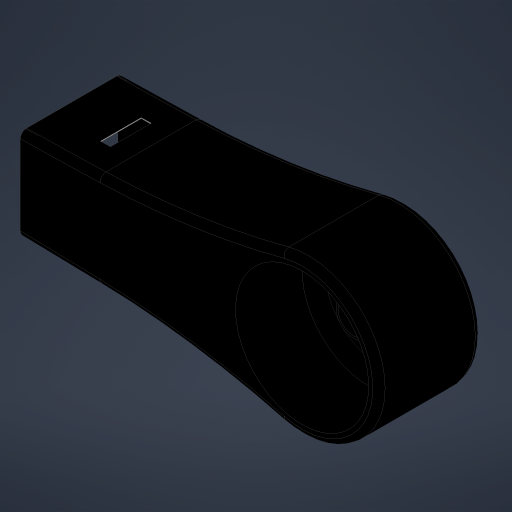
# Autodesk Inventor part: Arm
Saved by Autodesk Inventor 2023 (Build 270158000, 158)
## iProperties
Created: 2023-04-09
Part Number: Arm
Material: Generic
Document SubType Name: Modeling
Designer: vatdu
Density: 1 g/cm^3
Appearance: Default
Author: vatdu
Autodesk Inventor part; units mm, degrees
ref_plane "YZ Plane" through (0, 0, 0) normal (1, 0, 0) x (0, 1, 0)
ref_plane "XZ Plane" through (0, 0, 0) normal (0, 1, 0) x (-1, 0, 0)
ref_plane "XY Plane" through (0, 0, 0) normal (0, 0, 1) x (1, 0, 0)
sketch "Sketch1" plane through (0, 0, 0) normal (0, 0, 1) x (1, 0, 0)
  circle A0 centre (0, 0) radius 37.5
  line L0 (-37.5, 0.0313) -> (-137.5, 0.0313)
  line L1 (-137.5, 0.0313) -> (-137.5, -22.4687)
  line L2 (-137.5, -22.4687) -> (-137.5, 22.5313)
  line L3 (0, 0) -> (-26.5165, -26.5165)
  line L4 (0, 0) -> (37.5, 0) construction
  line L5 (-26.5165, -26.5165) -> (-26.5165, 26.5165)
  arc A1 (-137.5, 22.5313) -> (-26.5165, 26.5165) centre (-184.9263, 2890.6867) ccw
  arc A2 (-26.5165, -26.5165) -> (-137.5, -22.4687) centre (-183.0255, -2794.1927) ccw
  dimension "d0" = 75
  dimension "d15" = 100
  dimension "d16" = 22.5
  dimension "d17" = 45
  dimension "d18" = 37.5
  dimension "d19" = 135
  constraints: 12 end point, 6 point on circle, 3 centre point, 2 horizontal, 1 coincident, 1 equal length, 1 perpendicular, 1 point on line, 1 vertical
  measures "d0" diameter of A0
  measures "d15" distance of L0.start L0.end
  measures "d16" distance of L0.end L1.end
  measures "d17" distance of L1.end L2.end
  measures "d18" distance of L3.start L3.end
  measures "d19" angle of L3 L4
extrude "Extrusion1" add sketch "Sketch1" along normal blind 50
sketch "Sketch2" plane through (0, 0, 50) normal (0, 0, 1) x (0, 1, 0)
  circle A0 centre (0, 0) radius 32.5
  dimension "d3" = 65
  constraints: 1 centre point, 1 coincident
  measures "d3" diameter of A0
extrude "Extrusion2" cut sketch "Sketch2" against normal blind 40
sketch "Sketch3" plane through (0, 0, 10) normal (0, 0, 1) x (1, 0, 0)
  circle A0 centre (0, 0) radius 7.5
  circle A1 centre (0, 0) radius 8.5
  dimension "d6" = 15
  dimension "d7" = 17
  constraints: 2 centre point, 2 coincident
  measures "d6" diameter of A0
  measures "d7" diameter of A1
extrude "Extrusion3" add sketch "Sketch3" along normal blind 15
chamfer "Chamfer1" distance 24 distance2 10 1 edges at (-8.5, 0, 10) measured on face at (-9, 0, 10)
fillet "Fillet1" radius 10 1 edges at (-8.5, 0, 19.9999)
fillet "Fillet2" radius 5 2 edges at (-32.4999, 0, 10) (0, -32.5, 10)
fillet "Fillet5" radius 400 2 edges at (-26.5165, -26.5165, 25) (-26.5165, 26.5165, 25)
fillet "Fillet6" radius 3 10 edges at (-53.7386, 27.3358, 0) (-118.1043, 22.9176, 0) (37.5, -0.0111, 0) (-53.8089, -27.2963, 0) (-118.1658, -22.8537, 0) (-53.7386, 27.3358, 50) (37.5, -0.0111, 50) (-53.8089, -27.2963, 50) (-118.1658, -22.8537, 50) (-118.1043, 22.9176, 50)
sketch "Sketch5" plane through (-137.5, -19.4683, 0) normal (-1, 0, 0) x (0, 0, 1)
  line L0 (0, 19.4683) -> (2.5, 19.4683)
  line L1 (2.5, 19.4683) -> (2.5, -3.0317)
  line L2 (2.5, -3.0317) -> (47.5, -3.0317)
  ellipse E0 centre (47, -0.9067) end of major axis (50, -0.9067) minor radius 2.9986 (47, -3.9053) -> (50, -0.9067) ccw projected
  line L3 (47.5, -3.0317) -> (47.5, 41.9683)
  line L4 (47.5, 41.9683) -> (2.5, 41.9683)
  line L5 (2.5, 19.4683) -> (2.5, 41.9683)
  dimension "d29" = 2.5
  dimension "d30" = 45
  dimension "d31" = 90
  dimension "d32" = 45
  dimension "d33" = 90
  dimension "d34" = 45
  constraints: 10 end point, 2 vertical, 1 horizontal, 1 perpendicular, 1 point on line, 4 other
  measures "d29" distance of L0.start L0.end
  measures "d30" distance of L1.end L3.start
  measures "d31" angle to the sketch x axis of L1
  measures "d32" distance of L3.start L3.end
  measures "d33" angle to the sketch x axis of L3
  measures "d34" distance of L3.end L4.end
extrude "Extrusion5" cut sketch "Sketch5" against normal blind 35
sketch "Sketch6" plane through (0, 0, 0) normal (0, 0, -1) x (-1, 0, 0)
  circle A0 centre (0, 0) radius 25
  dimension "d37" = 50
  constraints: 1 centre point, 1 coincident
  measures "d37" diameter of A0
extrude "Extrusion6" add sketch "Sketch6" along normal blind 5
fillet "Fillet7" radius 2 1 edges at (25, 0, -5)
sketch "Sketch8" plane through (-137.5, 22.5, 2.5677) normal (0, -1, 0) x (1, 0, 0)
  line L0 (35, 44.9323) -> (35, -0.0677) projected
  line L1 (35, 22.4323) -> (29, 22.4323)
  line L2 (29, 22.4323) -> (29, 32.4323)
  line L3 (29, 32.4323) -> (24, 32.4323)
  line L4 (24, 32.4323) -> (24, 12.4323)
  line L5 (24, 12.4323) -> (29, 12.4323)
  line L6 (29, 12.4323) -> (29, 32.4323)
  point P0 (137.5, -2.5677)
  dimension "d47" = 6
  dimension "d48" = 10
  dimension "d49" = 5
  dimension "d50" = 20
  constraints: 12 end point, 2 horizontal, 2 parallel, 2 perpendicular, 1 midpoint
  measures "d47" distance of L1.start L1.end
  measures "d48" distance of L1.end L2.end
  measures "d49" distance of L5.end L4.end
  measures "d50" distance of L4.end L3.end
extrude "Extrusion8" cut sketch "Sketch8" against normal blind 6
equation "\"d51\" = d47"
body "Solid1"
